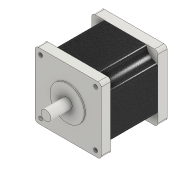
# Autodesk Inventor part: NEMA Motor-43
Saved by Autodesk Inventor 2020.1 (Build 241239000, 239)
## iProperties
Created: 2019-09-15
Part Number: NEMA Motor-43
Material: Generic
Document SubType Name: Modeling
Designer: thomastremblay
Density: 1 g/cm^3
Appearance: Steel
Author: thomastremblay
Autodesk Inventor part; units mm, degrees
ref_plane "YZ Plane" through (0, 0, 0) normal (1, 0, 0) x (0, 1, 0)
ref_plane "XZ Plane" through (0, 0, 0) normal (0, 1, 0) x (-1, 0, 0)
ref_plane "XY Plane" through (0, 0, 0) normal (0, 0, 1) x (1, 0, 0)
sketch "Sketch1" plane through (0, 0, 0) normal (0, 0, 1) x (1, 0, 0)
  circle A0 centre (0, 0) radius 27.7622
  line L0 (-53.34, -53.34) -> (53.34, -53.34)
  line L1 (53.34, -53.34) -> (53.34, 53.34)
  line L2 (53.34, 53.34) -> (-53.34, 53.34)
  line L3 (-53.34, 53.34) -> (-53.34, -53.34)
  line L4 (-53.34, -53.34) -> (53.34, 53.34) construction
  line L5 (53.34, -53.34) -> (-53.34, 53.34) construction
  circle A1 centre (0, 0) radius 7.9375
  line L6 (-44.45, -44.45) -> (44.45, -44.45) construction
  line L7 (44.45, -44.45) -> (44.45, 44.45) construction
  line L8 (44.45, 44.45) -> (-44.45, 44.45) construction
  line L9 (-44.45, 44.45) -> (-44.45, -44.45) construction
  line L10 (-44.45, -44.45) -> (44.45, 44.45) construction
  line L11 (44.45, -44.45) -> (-44.45, 44.45) construction
  dimension "Size" = 106.68
  dimension "pilot_dia" = 55.5244
  dimension "bolt_space" = 88.9
  dimension "shaft_dia" = 15.875
  constraints: 24 end point, 4 midpoint, 4 parallel, 3 perpendicular, 2 centre point, 2 coincident, 2 horizontal, 1 point on line
  measures "Size" distance of L0.end L1.end
  measures "pilot_dia" diameter of A0
  measures "bolt_space" distance of L6.end L7.end
  measures "shaft_dia" diameter of A1
extrude "Pilot" add sketch "Sketch1" along normal blind 1.5748 contours A0
extrude "Shaft" add sketch "Sketch1" along normal blind 36.068 contours A1
extrude "Extrusion3" add sketch "Sketch1" against normal blind 15.24 contours A0 | L3 L2 L1 L0 | A1
extrude "Extrusion4" add sketch "Sketch1" against normal blind 76.2 from surface at -15.24 separate body contours A0 | L3 L2 L1 L0 | A1
extrude "Extrusion5" add sketch "Sketch1" against normal blind 15.24 from surface at -91.44 separate body contours A0 | L3 L2 L1 L0 | A1
fillet "Fillet1" radius 17.78 4 edges at (-53.34, 53.34, -53.34) (-53.34, -53.34, -53.34) (53.34, -53.34, -53.34) (53.34, 53.34, -53.34) inverted yes
fillet "Fillet2" radius 5.08 16 edges at (-53.34, 53.34, -7.62) (-53.34, -53.34, -7.62) (53.34, -53.34, -7.62) (53.34, 53.34, -7.62) (-35.56, 53.34, -53.34) (53.34, -35.56, -53.34) (-53.34, 35.56, -53.34) (35.56, -53.34, -53.34) (-35.56, -53.34, -53.34) (-53.34, -35.56, -53.34) (35.56, 53.34, -53.34) (53.34, 35.56, -53.34) (-53.34, 53.34, -99.06) (53.34, 53.34, -99.06) (-53.34, -53.34, -99.06) (53.34, -53.34, -99.06)
hole "Hole1" at (44.45, 44.45, 0) at (44.45, -44.45, 0) at (-44.45, 44.45, 0) at (-44.45, -44.45, 0) direction (0, 0, -1) diameter 6.4008 depth 15.24 bodies 1 thread size "5/16-18 UNC" class "2B" standard "ANSI Unified Screw Threads"
body "Solid1"
body "Solid2"
body "Solid3"
